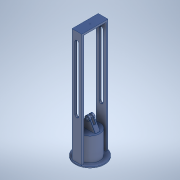
# Autodesk Inventor part: 2 nd link articulated
Saved by Autodesk Inventor 2020 (Build 240168000, 168)
## iProperties
Created: 2020-07-09
Part Number: 2 nd link articulated
Material: Generic
Document SubType Name: Modeling
Designer: Vikki
Density: 1 g/cm^3
Appearance: Flaked Satin - Blue
Mass: 58135.5 g
Surface Area: 41973.8 cm^2
Volume: 58135.5 cm^3
Author: Vikki
Autodesk Inventor part; units mm, degrees
ref_plane "YZ Plane" through (0, 0, 0) normal (1, 0, 0) x (0, 1, 0)
ref_plane "XZ Plane" through (0, 0, 0) normal (0, 1, 0) x (-1, 0, 0)
ref_plane "XY Plane" through (0, 0, 0) normal (0, 0, 1) x (1, 0, 0)
sketch "Sketch1" plane through (0, 0, 0) normal (0, 1, 0) x (-1, 0, 0)
  circle A0 centre (0, 0) radius 200
  circle A1 centre (0, 0) radius 175
  dimension "d0" = 400
  dimension "d1" = 350
  constraints: 2 centre point, 2 coincident
  measures "d0" diameter of A0
  measures "d1" diameter of A1
extrude "Extrusion1" add sketch "Sketch1" along normal blind 450
sketch "Sketch2" plane through (0, 450, 0) normal (0, 1, 0) x (1, 0, 0)
  circle A0 centre (0, 0) radius 200 projected
extrude "Extrusion2" add sketch "Sketch2" along normal blind 50
sketch "Sketch4" plane through (0, 0, 0) normal (0, 0, 1) x (1, 0, 0)
  circle A0 centre (0, 700) radius 25
  line L0 (200, 500) -> (-200, 500) projected
  circle A1 centre (0, 700) radius 50
  line L1 (0, 500) -> (160, 500)
  line L2 (160, 500) -> (50, 700)
  line L3 (0, 500) -> (-160, 500)
  line L4 (-160, 500) -> (-50, 700)
  point P0 (0, 0)
  dimension "d6" = 700
  dimension "d7" = 0
  dimension "d8" = 50
  dimension "d9" = 100
  dimension "d10" = 160
  dimension "d11" = 160
  constraints: 8 end point, 2 centre point, 2 coincident, 2 point on circle, 2 point on line, 1 midpoint
  measures "d6" distance of point (0, 700) point (0, 0)
  measures "d7" horizontal distance of point (0, 0) point (0, 700)
  measures "d8" diameter of A0
  measures "d9" diameter of A1
  measures "d10" distance of L1.start L1.end
  measures "d11" distance of L1.start L3.end
extrude "Extrusion3" add sketch "Sketch4" along normal mid plane 100 contours L0 L4 A1 L2
extrude "Extrusion4" add sketch "Sketch4" along normal mid plane 120 contours A1
ref_plane "Work Plane1" through (0, 900, 0) normal (0, 1, 0) x (1, 0, 0)
sketch "Sketch5" plane through (0, 900, 0) normal (0, 1, 0) x (1, 0, 0)
  line L0 (-93.2, -20) -> (93.2, -20)
  line L1 (93.2, -20) -> (93.2, 20)
  line L2 (93.2, 20) -> (-93.2, 20)
  line L3 (-93.2, 20) -> (-93.2, -20)
  line L4 (-93.2, -20) -> (93.2, 20) construction
  line L5 (93.2, -20) -> (-93.2, 20) construction
  point P0 (0, 0)
  dimension "d17" = 40
  constraints: 12 end point, 2 midpoint, 2 parallel, 1 horizontal, 1 perpendicular
  measures "d17" distance of L1.end L0.end
extrude "Extrusion5" cut sketch "Sketch5" against normal up to surface (400 mm away)
ref_plane "Work Plane2" through (0, 0, 0) normal (0, 1, 0) x (1, 0, 0)
sketch "Sketch6" plane through (0, 0, 0) normal (0, 1, 0) x (1, 0, 0)
  circle A0 centre (0, 0) radius 175 projected
  circle A1 centre (0, 0) radius 300
  dimension "d20" = 600
  constraints: 1 centre point, 1 coincident
  measures "d20" diameter of A1
extrude "Extrusion6" add sketch "Sketch6" along normal blind 20
sketch "Sketch7" plane through (0, 20, 0) normal (0, 1, 0) x (1, 0, 0)
  line L0 (100, -270) -> (-100, -270)
  line L1 (-100, -270) -> (-100, -230)
  line L2 (-100, -230) -> (100, -230)
  line L3 (100, -230) -> (100, -270)
  circle A0 centre (0, 0) radius 300 projected
  line L4 (59.8152, 0) -> (-33.1848, 0)
  line L5 (100, 270) -> (-100, 270)
  line L6 (-100, 270) -> (-100, 230)
  line L7 (-100, 230) -> (100, 230)
  line L8 (100, 230) -> (100, 270)
  dimension "d23" = 200
  dimension "d24" = 100
  dimension "d25" = 40
  dimension "d26" = 270
  dimension "d27" = 0
  constraints: 18 end point, 4 symmetric about line, 2 horizontal, 2 parallel, 1 perpendicular
  measures "d23" distance of L1.end L2.end
  measures "d24" distance from line of point (0, 0) L1
  measures "d25" distance of L0.end L1.end
  measures "d26" distance from line of L0 A0.centre
  measures "d27" distance from line of L4 point (0, 0)
extrude "Extrusion7" add sketch "Sketch7" along normal blind 2300 contours L0 L1 L2 L3 | L8 L7 L6 L5
sketch "Sketch8" plane through (0, 2320, 0) normal (0, 1, 0) x (1, 0, 0)
  line L0 (-100, -270) -> (100, -270) projected
  line L1 (-100, 270) -> (-100, 230) projected
  line L2 (-100, -270) -> (-100, 270)
  line L3 (100, -270) -> (100, -230) projected
  line L4 (100, 270) -> (-100, 270) projected
  line L5 (100, -270) -> (100, 270)
  point P0 (0, 0)
  point P1 (-100, 230)
  constraints: 4 end point, 1 collinear, 1 perpendicular
extrude "Extrusion8" add sketch "Sketch8" along normal blind 40
sketch "Sketch9" plane through (100, 20, -270) normal (0, 0, -1) x (-1, 0, 0)
  line L0 (100, 840) -> (100, 2140) construction
  line L1 (140, 840) -> (140, 2140)
  line L2 (60, 2140) -> (60, 840)
  arc A0 (60, 840) -> (140, 840) centre (100, 840) ccw
  arc A1 (140, 2140) -> (60, 2140) centre (100, 2140) ccw
  line L3 (0, 0) -> (0, 2340) projected
  line L4 (200, 0) -> (200, 2340) projected
  line L5 (0, 2340) -> (200, 2340) projected
  point P0 (100, -20)
  point P1 (100, 1490)
  dimension "d32" = 60
  dimension "d33" = 60
  dimension "d34" = 40
  dimension "d35" = 1300
  dimension "d36" = 200
  constraints: 8 end point, 4 point on circle, 4 tangent, 2 centre point, 1 midpoint, 1 parallel, 1 vertical
  measures "d32" distance between parallel lines of L2 L3
  measures "d33" distance between parallel lines of L4 L1
  measures "d34" radius of A1
  measures "d35" distance of L0.start L0.end
  measures "d36" distance from line of L5 L0.end
extrude "Extrusion9" cut sketch "Sketch9" against normal up to surface (540 mm away)
sketch "Sketch10" plane through (0, 2360, 0) normal (0, 1, 0) x (1, 0, 0)
  circle A0 centre (0, 0) radius 8.25
  point P0 (0, 0)
  dimension "d39" = 16.5
  constraints: 1 centre point, 1 coincident
  measures "d39" diameter of A0
extrude "Extrusion10" cut sketch "Sketch10" against normal up to surface (40 mm away)
ref_plane "Work Plane5" through (0, 750, 0) normal (0, -1, 0) x (1, 0, 0)
ref_plane "Work Plane4" through (-1699.7896, 400, 26.7465) normal (0, -1, 0) x (-0.9998762, 0, 0.0157332)
fillet "Fillet2" radius 3 15 edges at (-50, 700, -60) (-50, 700, 60) (0, 750, 20) (0, 750, -20) (71.6, 660.7273, -20) (105, 600, -50) (71.6, 660.7273, 20) (93.2, 621.4545, 0) (105, 600, 50) (160, 500, 0) (-93.2, 621.4545, 0) (-71.6, 660.7273, -20) (-71.6, 660.7273, 20) (-105, 600, 50) (-105, 600, -50)
equation "\"d11\" = d10"
equation "\"d33\" = d32"
body "Solid1"
